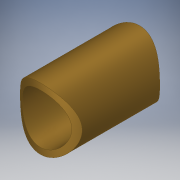
# Autodesk Inventor part: Piston Bushing
Saved by Autodesk Inventor 2018 (Build 220112000, 112)
## iProperties
Created: 2017-09-20
Part Number: Piston Bushing
Material: Generic
Document SubType Name: Modeling
Designer: Intel
Density: 1 g/cm^3
Appearance: Brass - Satin
Author: Intel
Autodesk Inventor part; units mm, degrees
ref_plane "YZ Plane" through (0, 0, 0) normal (1, 0, 0) x (0, 1, 0)
ref_plane "XZ Plane" through (0, 0, 0) normal (0, 1, 0) x (-1, 0, 0)
ref_plane "XY Plane" through (0, 0, 0) normal (0, 0, 1) x (1, 0, 0)
sketch "Sketch1" plane through (0, 0, 0) normal (0, 0, 1) x (1, 0, 0)
  circle A0 centre (0, 0) radius 3.9624
  circle A1 centre (0, 0) radius 3.175
  dimension "d0" = 7.9248
  dimension "d1" = 6.35
  constraints: 2 centre point, 2 coincident
  measures "d0" diameter of A0
  measures "d1" diameter of A1
extrude "Extrusion1" add sketch "Sketch1" along normal blind 12.7
sketch "Sketch2" plane through (0, 0, 0) normal (0, 1, 0) x (-1, 0, 0)
  circle A0 centre (0, 6.35) radius 6.35
  line L0 (-3.9624, 0) -> (3.9624, 0) projected
  line L1 (3.9624, 12.7) -> (-3.9624, 12.7) projected
  line L2 (3.9624, 0) -> (3.9624, 12.7) projected
  line L3 (3.9624, 0) -> (3.9624, 12.7) projected
  circle A1 centre (0, 6.35) radius 9.525
  point P0 (0, 0)
  dimension "d4" = 12.7
  dimension "d5" = 3.9624
  dimension "d6" = 19.05
  constraints: 2 centre point, 1 coincident, 1 tangent
  measures "d4" diameter of A0
  measures "d5" distance from line of L2 A0.centre
  measures "d6" diameter of A1
extrude "Extrusion2" cut sketch "Sketch2" along normal mid plane 12.7 contours A0 L1 L2 | L2 L0 A0 | A1
body "Solid1"
